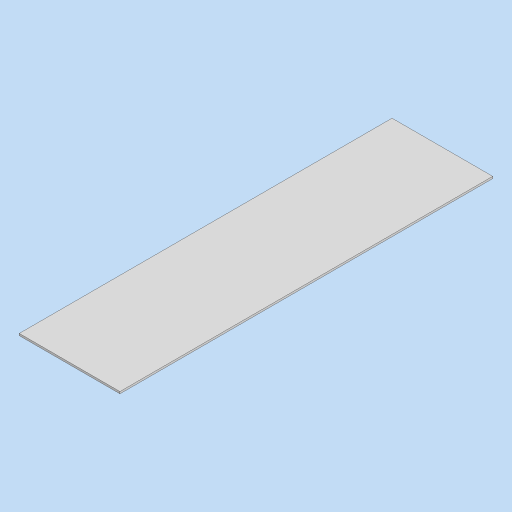
# Autodesk Inventor part: BatteryBoxSheetMetal
Saved by Autodesk Inventor 2023 (Build 270158000, 158)
## iProperties
Created: 2023-01-22
Part Number: BatteryBoxSheetMetal
Material: Generic
Document SubType Name: Sheet Metal
Designer: asach
Density: 1 g/cm^3
Sheet Metal Rule: Default
Appearance: Default
Author: asach
Autodesk Inventor part; units mm, degrees
ref_plane "YZ Plane" through (0, 0, 0) normal (1, 0, 0) x (0, 1, 0)
ref_plane "XZ Plane" through (0, 0, 0) normal (0, 1, 0) x (-1, 0, 0)
ref_plane "XY Plane" through (0, 0, 0) normal (0, 0, 1) x (1, 0, 0)
sketch "Sketch1" plane through (0, 0, 0) normal (0, 1, 0) x (-1, 0, 0)
  line L0 (0, 0) -> (162, 0)
  line L1 (162, 0) -> (162, -600)
  line L2 (162, -600) -> (0, -600)
  line L3 (0, -600) -> (0, 0)
  dimension "d0" = 162
  dimension "d1" = 600
  constraints: 8 end point, 2 parallel, 1 horizontal, 1 perpendicular
  measures "d0" distance of L1.end L2.end
  measures "d1" distance of L0.end L1.end
extrude "Extrusion1" add sketch "Sketch1" along normal blind 3.175
equation "\"d0\" = batteryBoxWidth"
equation "\"d1\" = batteryBoxLength"
equation "\"d2\" = sheetMetalThickness"
equation "\"BendRadius\" = Thickness"
equation "\"BendReliefWidth\" = Thickness"
equation "\"BendReliefDepth\" = 0.5 * Thickness"
equation "\"CornerReliefSize\" = 4 * Thickness"
equation "\"MinimumRemnant\" = 2 * Thickness"
equation "\"TransitionRadius\" = BendRadius"
equation "\"JacobiRadiusSize\" = BendRadius"
equation "\"GapSize\" = Thickness"
equation "\"tolerance\" = 0.2"
equation "\"cellSpacing\" = 1"
equation "\"screwDiameter\" = 5"
equation "\"baseThickness\" = 7"
equation "\"tabThickness\" = 0.8"
equation "\"batteryBoxWidth\" = 162"
equation "\"batteryBoxLength\" = 600"
equation "\"sheetMetalThickness\" = 3.175"
equation "\"Thickness\" = 3.048"
body "Solid1"
